Autodesk Fusion 360 part; units mm, degrees
(part 3 of 5)
  spline S30 degree 5 poles (2.192, 23.3898) (2.1931, 23.4016) (2.195, 23.4251) (2.1969, 23.4604) (2.1976, 23.5076) (2.1961, 23.5666) (2.1928, 23.6257) (2.1885, 23.6849) (2.1835, 23.7441) (2.1781, 23.8033) (2.1724, 23.8626) (2.166, 23.9218) (2.159, 23.9811) (2.151, 24.0404) (2.1423, 24.0996) (2.1327, 24.1589) (2.1224, 24.2182) (2.1116, 24.2775) (2.1003, 24.3368) (2.0885, 24.396) (2.0763, 24.4553) (2.0635, 24.5145) (2.0503, 24.5737) (2.0365, 24.6329) (2.0221, 24.6921) (2.0073, 24.7513) (1.992, 24.8104) (1.9762, 24.8696) (1.96, 24.9287) (1.9433, 24.9877) (1.9262, 25.0468) (1.9087, 25.1058) (1.8908, 25.1648) (1.8724, 25.2237) (1.8536, 25.2826) (1.8344, 25.3415) (1.8148, 25.4004) (1.7947, 25.4592) (1.7743, 25.518) (1.7535, 25.5767) (1.7323, 25.6354) (1.7108, 25.694) (1.6888, 25.7526) (1.6665, 25.8112) (1.6438, 25.8697) (1.6207, 25.9282) (1.5972, 25.9866) (1.5734, 26.045) (1.5493, 26.1034) (1.5248, 26.1616) (1.4999, 26.2199) (1.4747, 26.2781) (1.4491, 26.3362) (1.4232, 26.3943) (1.3969, 26.4523) (1.3704, 26.5102) (1.3434, 26.5682) (1.3162, 26.626) (1.2886, 26.6838) (1.2606, 26.7415) (1.2324, 26.7992) (1.2038, 26.8568) (1.1749, 26.9144) (1.1457, 26.9719) (1.1161, 27.0293) (1.0863, 27.0866) (1.0561, 27.1439) (1.0256, 27.2012) (0.9948, 27.2583) (0.9637, 27.3154) (0.9323, 27.3725) (0.9069, 27.418) (0.8877, 27.4522) (0.8749, 27.4749) (0.8685, 27.4863) knots 0 0 0 0 0 0 0.01428571 0.02857143 0.04285714 0.05714286 0.07142857 0.08571429 0.1 0.11428571 0.12857143 0.14285714 0.15714286 0.17142857 0.18571429 0.2 0.21428571 0.22857143 0.24285714 0.25714286 0.27142857 0.28571429 0.3 0.31428571 0.32857143 0.34285714 0.35714286 0.37142857 0.38571429 0.4 0.41428571 0.42857143 0.44285714 0.45714286 0.47142857 0.48571429 0.5 0.51428571 0.52857143 0.54285714 0.55714286 0.57142857 0.58571429 0.6 0.61428571 0.62857143 0.64285714 0.65714286 0.67142857 0.68571429 0.7 0.71428571 0.72857143 0.74285714 0.75714286 0.77142857 0.78571429 0.8 0.81428571 0.82857143 0.84285714 0.85714286 0.87142857 0.88571429 0.9 0.91428571 0.92857143 0.94285714 0.95714286 0.97142857 0.98571429 1 1 1 1 1 1
  arc A62 (0.8685, 27.4863) -> (-0.8685, 27.4863) centre (0, 0) ccw
  spline S31 degree 5 poles (-0.8685, 27.4863) (-0.8749, 27.4749) (-0.8877, 27.4522) (-0.9069, 27.418) (-0.9323, 27.3725) (-0.9637, 27.3154) (-0.9948, 27.2583) (-1.0256, 27.2012) (-1.0561, 27.1439) (-1.0863, 27.0866) (-1.1161, 27.0293) (-1.1457, 26.9719) (-1.1749, 26.9144) (-1.2038, 26.8568) (-1.2324, 26.7992) (-1.2606, 26.7415) (-1.2886, 26.6838) (-1.3162, 26.626) (-1.3434, 26.5682) (-1.3704, 26.5102) (-1.3969, 26.4523) (-1.4232, 26.3943) (-1.4491, 26.3362) (-1.4747, 26.2781) (-1.4999, 26.2199) (-1.5248, 26.1616) (-1.5493, 26.1034) (-1.5734, 26.045) (-1.5972, 25.9866) (-1.6207, 25.9282) (-1.6438, 25.8697) (-1.6665, 25.8112) (-1.6888, 25.7526) (-1.7108, 25.694) (-1.7323, 25.6354) (-1.7535, 25.5767) (-1.7743, 25.518) (-1.7947, 25.4592) (-1.8148, 25.4004) (-1.8344, 25.3415) (-1.8536, 25.2826) (-1.8724, 25.2237) (-1.8908, 25.1648) (-1.9087, 25.1058) (-1.9262, 25.0468) (-1.9433, 24.9877) (-1.96, 24.9287) (-1.9762, 24.8696) (-1.992, 24.8104) (-2.0073, 24.7513) (-2.0221, 24.6921) (-2.0365, 24.6329) (-2.0503, 24.5737) (-2.0635, 24.5145) (-2.0763, 24.4553) (-2.0885, 24.396) (-2.1003, 24.3368) (-2.1116, 24.2775) (-2.1224, 24.2182) (-2.1327, 24.1589) (-2.1423, 24.0996) (-2.151, 24.0404) (-2.159, 23.9811) (-2.166, 23.9218) (-2.1724, 23.8626) (-2.1781, 23.8033) (-2.1835, 23.7441) (-2.1885, 23.6849) (-2.1928, 23.6257) (-2.1961, 23.5666) (-2.1976, 23.5076) (-2.1969, 23.4604) (-2.195, 23.4251) (-2.1931, 23.4016) (-2.192, 23.3898) knots -1 -1 -1 -1 -1 -1 -0.98571429 -0.97142857 -0.95714286 -0.94285714 -0.92857143 -0.91428571 -0.9 -0.88571429 -0.87142857 -0.85714286 -0.84285714 -0.82857143 -0.81428571 -0.8 -0.78571429 -0.77142857 -0.75714286 -0.74285714 -0.72857143 -0.71428571 -0.7 -0.68571429 -0.67142857 -0.65714286 -0.64285714 -0.62857143 -0.61428571 -0.6 -0.58571429 -0.57142857 -0.55714286 -0.54285714 -0.52857143 -0.51428571 -0.5 -0.48571429 -0.47142857 -0.45714286 -0.44285714 -0.42857143 -0.41428571 -0.4 -0.38571429 -0.37142857 -0.35714286 -0.34285714 -0.32857143 -0.31428571 -0.3 -0.28571429 -0.27142857 -0.25714286 -0.24285714 -0.22857143 -0.21428571 -0.2 -0.18571429 -0.17142857 -0.15714286 -0.14285714 -0.12857143 -0.11428571 -0.1 -0.08571429 -0.07142857 -0.05714286 -0.04285714 -0.02857143 -0.01428571 0 0 0 0 0 0
  line L31 (-2.192, 23.3898) -> (-2.1396, 22.8267)
  arc A63 (-2.9987, 21.7434) -> (-2.1396, 22.8267) centre (-3.1353, 22.734) ccw
  arc A64 (-2.9987, 21.7434) -> (-3.8672, 21.6058) centre (0, 0) ccw
  arc A65 (-5.019, 22.3707) -> (-3.8672, 21.6058) centre (-4.0434, 22.5902) ccw
  line L32 (-5.019, 22.3707) -> (-5.1431, 22.9224)
  spline S32 degree 5 poles (-5.1431, 22.9224) (-5.1457, 22.9339) (-5.1512, 22.9569) (-5.1603, 22.9911) (-5.1742, 23.0361) (-5.1939, 23.0918) (-5.2153, 23.147) (-5.2377, 23.2019) (-5.2607, 23.2567) (-5.2841, 23.3114) (-5.3079, 23.3659) (-5.3322, 23.4203) (-5.3573, 23.4745) (-5.3831, 23.5284) (-5.4098, 23.5821) (-5.4372, 23.6355) (-5.4653, 23.6888) (-5.4939, 23.7418) (-5.523, 23.7947) (-5.5525, 23.8474) (-5.5824, 23.9) (-5.6129, 23.9523) (-5.6438, 24.0046) (-5.6752, 24.0566) (-5.7071, 24.1085) (-5.7395, 24.1602) (-5.7724, 24.2117) (-5.8056, 24.263) (-5.8393, 24.3142) (-5.8734, 24.3653) (-5.9079, 24.4161) (-5.9428, 24.4668) (-5.9781, 24.5174) (-6.0138, 24.5678) (-6.0499, 24.618) (-6.0864, 24.6681) (-6.1232, 24.718) (-6.1604, 24.7677) (-6.198, 24.8173) (-6.2359, 24.8667) (-6.2742, 24.916) (-6.3129, 24.9651) (-6.3519, 25.0141) (-6.3912, 25.0629) (-6.4309, 25.1115) (-6.4709, 25.16) (-6.5112, 25.2083) (-6.5519, 25.2565) (-6.5929, 25.3045) (-6.6343, 25.3524) (-6.6759, 25.4001) (-6.7179, 25.4476) (-6.7601, 25.495) (-6.8027, 25.5422) (-6.8456, 25.5893) (-6.8888, 25.6362) (-6.9323, 25.683) (-6.9761, 25.7296) (-7.0202, 25.776) (-7.0646, 25.8223) (-7.1093, 25.8684) (-7.1543, 25.9144) (-7.1996, 25.9602) (-7.2452, 26.0058) (-7.291, 26.0513) (-7.3371, 26.0966) (-7.3835, 26.1418) (-7.4302, 26.1868) (-7.4772, 26.2316) (-7.5244, 26.2763) (-7.5719, 26.3208) (-7.6101, 26.3563) (-7.6389, 26.3829) (-7.6581, 26.4006) (-7.6678, 26.4094) knots 0 0 0 0 0 0 0.01428571 0.02857143 0.04285714 0.05714286 0.07142857 0.08571429 0.1 0.11428571 0.12857143 0.14285714 0.15714286 0.17142857 0.18571429 0.2 0.21428571 0.22857143 0.24285714 0.25714286 0.27142857 0.28571429 0.3 0.31428571 0.32857143 0.34285714 0.35714286 0.37142857 0.38571429 0.4 0.41428571 0.42857143 0.44285714 0.45714286 0.47142857 0.48571429 0.5 0.51428571 0.52857143 0.54285714 0.55714286 0.57142857 0.58571429 0.6 0.61428571 0.62857143 0.64285714 0.65714286 0.67142857 0.68571429 0.7 0.71428571 0.72857143 0.74285714 0.75714286 0.77142857 0.78571429 0.8 0.81428571 0.82857143 0.84285714 0.85714286 0.87142857 0.88571429 0.9 0.91428571 0.92857143 0.94285714 0.95714286 0.97142857 0.98571429 1 1 1 1 1 1
  arc A66 (-7.6678, 26.4094) -> (-9.3197, 25.8726) centre (0, 0) ccw
  spline S33 degree 5 poles (-9.3197, 25.8726) (-9.3223, 25.8598) (-9.3275, 25.8342) (-9.3352, 25.7958) (-9.3452, 25.7447) (-9.3575, 25.6807) (-9.3694, 25.6168) (-9.381, 25.5529) (-9.3924, 25.4891) (-9.4033, 25.4253) (-9.414, 25.3615) (-9.4244, 25.2977) (-9.4344, 25.234) (-9.4441, 25.1704) (-9.4535, 25.1067) (-9.4625, 25.0432) (-9.4712, 24.9796) (-9.4796, 24.9161) (-9.4877, 24.8527) (-9.4954, 24.7893) (-9.5028, 24.7259) (-9.5098, 24.6626) (-9.5165, 24.5994) (-9.5229, 24.5362) (-9.5289, 24.4731) (-9.5345, 24.41) (-9.5398, 24.347) (-9.5448, 24.2841) (-9.5494, 24.2212) (-9.5536, 24.1584) (-9.5575, 24.0956) (-9.561, 24.033) (-9.5642, 23.9704) (-9.5669, 23.9078) (-9.5693, 23.8454) (-9.5713, 23.783) (-9.573, 23.7207) (-9.5742, 23.6585) (-9.5751, 23.5964) (-9.5756, 23.5344) (-9.5756, 23.4724) (-9.5753, 23.4106) (-9.5746, 23.3488) (-9.5734, 23.2872) (-9.5718, 23.2257) (-9.5698, 23.1642) (-9.5674, 23.1029) (-9.5646, 23.0417) (-9.5613, 22.9806) (-9.5576, 22.9196) (-9.5535, 22.8587) (-9.5488, 22.798) (-9.5436, 22.7374) (-9.5379, 22.677) (-9.5318, 22.6167) (-9.5251, 22.5566) (-9.518, 22.4966) (-9.5104, 22.4367) (-9.5024, 22.377) (-9.4938, 22.3175) (-9.4846, 22.2581) (-9.4746, 22.199) (-9.4638, 22.1402) (-9.4523, 22.0817) (-9.44, 22.0233) (-9.4272, 21.9652) (-9.414, 21.9072) (-9.4004, 21.8494) (-9.3863, 21.7918) (-9.3711, 21.7346) (-9.3543, 21.6779) (-9.339, 21.6333) (-9.3263, 21.6003) (-9.3173, 21.5785) (-9.3126, 21.5677) knots -1 -1 -1 -1 -1 -1 -0.98571429 -0.97142857 -0.95714286 -0.94285714 -0.92857143 -0.91428571 -0.9 -0.88571429 -0.87142857 -0.85714286 -0.84285714 -0.82857143 -0.81428571 -0.8 -0.78571429 -0.77142857 -0.75714286 -0.74285714 -0.72857143 -0.71428571 -0.7 -0.68571429 -0.67142857 -0.65714286 -0.64285714 -0.62857143 -0.61428571 -0.6 -0.58571429 -0.57142857 -0.55714286 -0.54285714 -0.52857143 -0.51428571 -0.5 -0.48571429 -0.47142857 -0.45714286 -0.44285714 -0.42857143 -0.41428571 -0.4 -0.38571429 -0.37142857 -0.35714286 -0.34285714 -0.32857143 -0.31428571 -0.3 -0.28571429 -0.27142857 -0.25714286 -0.24285714 -0.22857143 -0.21428571 -0.2 -0.18571429 -0.17142857 -0.15714286 -0.14285714 -0.12857143 -0.11428571 -0.1 -0.08571429 -0.07142857 -0.05714286 -0.04285714 -0.02857143 -0.01428571 0 0 0 0 0 0
  line L33 (-9.3126, 21.5677) -> (-9.0887, 21.0483)
  arc A67 (-9.571, 19.7526) -> (-9.0887, 21.0483) centre (-10.007, 20.6525) ccw
  arc A68 (-9.571, 19.7526) -> (-10.3545, 19.3534) centre (0, 0) ccw
  arc A69 (-11.6862, 19.7248) -> (-10.3545, 19.3534) centre (-10.8262, 20.2351) ccw
  line L34 (-11.6862, 19.7248) -> (-11.9748, 20.2112)
  spline S34 degree 5 poles (-11.9748, 20.2112) (-11.9808, 20.2214) (-11.9931, 20.2415) (-12.0124, 20.2712) (-12.0395, 20.3098) (-12.0754, 20.3566) (-12.1128, 20.4025) (-12.1511, 20.4478) (-12.1899, 20.4928) (-12.2291, 20.5376) (-12.2686, 20.5821) (-12.3085, 20.6263) (-12.3491, 20.6701) (-12.3903, 20.7134) (-12.4323, 20.7562) (-12.4749, 20.7985) (-12.518, 20.8405) (-12.5616, 20.8821) (-12.6056, 20.9234) (-12.65, 20.9644) (-12.6947, 21.0051) (-12.7398, 21.0456) (-12.7854, 21.0857) (-12.8313, 21.1255) (-12.8777, 21.1649) (-12.9245, 21.2041) (-12.9717, 21.2429) (-13.0192, 21.2815) (-13.0671, 21.3198) (-13.1152, 21.3577) (-13.1638, 21.3955) (-13.2126, 21.4329) (-13.2618, 21.4701) (-13.3113, 21.507) (-13.3612, 21.5436) (-13.4113, 21.5799) (-13.4618, 21.616) (-13.5126, 21.6518) (-13.5636, 21.6874) (-13.615, 21.7227) (-13.6666, 21.7577) (-13.7185, 21.7925) (-13.7708, 21.827) (-13.8233, 21.8612) (-13.876, 21.8952) (-13.9291, 21.929) (-13.9824, 21.9625) (-14.0359, 21.9957) (-14.0898, 22.0287) (-14.1439, 22.0615) (-14.1982, 22.0939) (-14.2528, 22.1262) (-14.3077, 22.1582) (-14.3628, 22.1899) (-14.4181, 22.2215) (-14.4737, 22.2527) (-14.5295, 22.2837) (-14.5856, 22.3145) (-14.6419, 22.345) (-14.6984, 22.3753) (-14.7552, 22.4054) (-14.8121, 22.4352) (-14.8694, 22.4648) (-14.9268, 22.4941) (-14.9844, 22.5232) (-15.0423, 22.5521) (-15.1004, 22.5807) (-15.1587, 22.6091) (-15.2172, 22.6372) (-15.276, 22.6651) (-15.3349, 22.6928) (-15.3822, 22.7147) (-15.4178, 22.7311) (-15.4415, 22.7419) (-15.4534, 22.7473) knots 0 0 0 0 0 0 0.01428571 0.02857143 0.04285714 0.05714286 0.07142857 0.08571429 0.1 0.11428571 0.12857143 0.14285714 0.15714286 0.17142857 0.18571429 0.2 0.21428571 0.22857143 0.24285714 0.25714286 0.27142857 0.28571429 0.3 0.31428571 0.32857143 0.34285714 0.35714286 0.37142857 0.38571429 0.4 0.41428571 0.42857143 0.44285714 0.45714286 0.47142857 0.48571429 0.5 0.51428571 0.52857143 0.54285714 0.55714286 0.57142857 0.58571429 0.6 0.61428571 0.62857143 0.64285714 0.65714286 0.67142857 0.68571429 0.7 0.71428571 0.72857143 0.74285714 0.75714286 0.77142857 0.78571429 0.8 0.81428571 0.82857143 0.84285714 0.85714286 0.87142857 0.88571429 0.9 0.91428571 0.92857143 0.94285714 0.95714286 0.97142857 0.98571429 1 1 1 1 1 1
  arc A70 (-15.4534, 22.7473) -> (-16.8586, 21.7264) centre (0, 0) ccw
  spline S35 degree 5 poles (-16.8586, 21.7264) (-16.8572, 21.7134) (-16.8542, 21.6875) (-16.8496, 21.6486) (-16.8434, 21.5968) (-16.8353, 21.5322) (-16.8269, 21.4677) (-16.8182, 21.4034) (-16.8092, 21.3392) (-16.7999, 21.2751) (-16.7904, 21.2111) (-16.7805, 21.1473) (-16.7704, 21.0836) (-16.7599, 21.02) (-16.7492, 20.9566) (-16.7382, 20.8934) (-16.7268, 20.8302) (-16.7152, 20.7673) (-16.7032, 20.7044) (-16.691, 20.6418) (-16.6784, 20.5792) (-16.6656, 20.5169) (-16.6524, 20.4547) (-16.6389, 20.3926) (-16.6251, 20.3307) (-16.611, 20.269) (-16.5966, 20.2074) (-16.5818, 20.146) (-16.5668, 20.0848) (-16.5514, 20.0238) (-16.5357, 19.9629) (-16.5197, 19.9022) (-16.5033, 19.8417) (-16.4866, 19.7814) (-16.4696, 19.7212) (-16.4522, 19.6613) (-16.4345, 19.6015) (-16.4165, 19.542) (-16.3981, 19.4826) (-16.3794, 19.4235) (-16.3604, 19.3646) (-16.3409, 19.3059) (-16.3211, 19.2474) (-16.301, 19.1891) (-16.2805, 19.1311) (-16.2596, 19.0732) (-16.2383, 19.0157) (-16.2167, 18.9583) (-16.1948, 18.9012) (-16.1724, 18.8444) (-16.1496, 18.7878) (-16.1264, 18.7315) (-16.1028, 18.6754) (-16.0787, 18.6197) (-16.0542, 18.5643) (-16.0293, 18.5092) (-16.004, 18.4543) (-15.9783, 18.3997) (-15.9522, 18.3454) (-15.9256, 18.2914) (-15.8985, 18.2378) (-15.8708, 18.1847) (-15.8424, 18.1321) (-15.8132, 18.08) (-15.7835, 18.0283) (-15.7534, 17.977) (-15.7229, 17.9259) (-15.6921, 17.8751) (-15.6609, 17.8247) (-15.6288, 17.775) (-15.5953, 17.7263) (-15.567, 17.6886) (-15.5447, 17.6611) (-15.5294, 17.6432) (-15.5216, 17.6343) knots -1 -1 -1 -1 -1 -1 -0.98571429 -0.97142857 -0.95714286 -0.94285714 -0.92857143 -0.91428571 -0.9 -0.88571429 -0.87142857 -0.85714286 -0.84285714 -0.82857143 -0.81428571 -0.8 -0.78571429 -0.77142857 -0.75714286 -0.74285714 -0.72857143 -0.71428571 -0.7 -0.68571429 -0.67142857 -0.65714286 -0.64285714 -0.62857143 -0.61428571 -0.6 -0.58571429 -0.57142857 -0.55714286 -0.54285714 -0.52857143 -0.51428571 -0.5 -0.48571429 -0.47142857 -0.45714286 -0.44285714 -0.42857143 -0.41428571 -0.4 -0.38571429 -0.37142857 -0.35714286 -0.34285714 -0.32857143 -0.31428571 -0.3 -0.28571429 -0.27142857 -0.25714286 -0.24285714 -0.22857143 -0.21428571 -0.2 -0.18571429 -0.17142857 -0.15714286 -0.14285714 -0.12857143 -0.11428571 -0.1 -0.08571429 -0.07142857 -0.05714286 -0.04285714 -0.02857143 -0.01428571 0 0 0 0 0 0
  line L35 (-15.5216, 17.6343) -> (-15.1482, 17.2096)
  arc A71 (-15.2064, 15.8282) -> (-15.1482, 17.2096) centre (-15.8992, 16.5493) ccw
  arc A72 (-15.2064, 15.8282) -> (-15.8282, 15.2064) centre (0, 0) ccw
  arc A73 (-17.2096, 15.1482) -> (-15.8282, 15.2064) centre (-16.5493, 15.8992) ccw
  line L36 (-17.2096, 15.1482) -> (-17.6343, 15.5216)
  spline S36 degree 5 poles (-17.6343, 15.5216) (-17.6432, 15.5294) (-17.6611, 15.5447) (-17.6886, 15.567) (-17.7263, 15.5953) (-17.775, 15.6288) (-17.8247, 15.6609) (-17.8751, 15.6921) (-17.9259, 15.7229) (-17.977, 15.7534) (-18.0283, 15.7835) (-18.08, 15.8132) (-18.1321, 15.8424) (-18.1847, 15.8708) (-18.2378, 15.8985) (-18.2914, 15.9256) (-18.3454, 15.9522) (-18.3997, 15.9783) (-18.4543, 16.004) (-18.5092, 16.0293) (-18.5643, 16.0542) (-18.6197, 16.0787) (-18.6754, 16.1028) (-18.7315, 16.1264) (-18.7878, 16.1496) (-18.8444, 16.1724) (-18.9012, 16.1948) (-18.9583, 16.2167) (-19.0157, 16.2383) (-19.0732, 16.2596) (-19.1311, 16.2805) (-19.1891, 16.301) (-19.2474, 16.3211) (-19.3059, 16.3409) (-19.3646, 16.3604) (-19.4235, 16.3794) (-19.4826, 16.3981) (-19.542, 16.4165) (-19.6015, 16.4345) (-19.6613, 16.4522) (-19.7212, 16.4696) (-19.7814, 16.4866) (-19.8417, 16.5033) (-19.9022, 16.5197) (-19.9629, 16.5357) (-20.0238, 16.5514) (-20.0848, 16.5668) (-20.146, 16.5818) (-20.2074, 16.5966) (-20.269, 16.611) (-20.3307, 16.6251) (-20.3926, 16.6389) (-20.4547, 16.6524) (-20.5169, 16.6656) (-20.5792, 16.6784) (-20.6418, 16.691) (-20.7044, 16.7032) (-20.7673, 16.7152) (-20.8302, 16.7268) (-20.8934, 16.7382) (-20.9566, 16.7492) (-21.02, 16.7599) (-21.0836, 16.7704) (-21.1473, 16.7805) (-21.2111, 16.7904) (-21.2751, 16.7999) (-21.3392, 16.8092) (-21.4034, 16.8182) (-21.4677, 16.8269) (-21.5322, 16.8353) (-21.5968, 16.8434) (-21.6486, 16.8496) (-21.6875, 16.8542) (-21.7134, 16.8572) (-21.7264, 16.8586) knots 0 0 0 0 0 0 0.01428571 0.02857143 0.04285714 0.05714286 0.07142857 0.08571429 0.1 0.11428571 0.12857143 0.14285714 0.15714286 0.17142857 0.18571429 0.2 0.21428571 0.22857143 0.24285714 0.25714286 0.27142857 0.28571429 0.3 0.31428571 0.32857143 0.34285714 0.35714286 0.37142857 0.38571429 0.4 0.41428571 0.42857143 0.44285714 0.45714286 0.47142857 0.48571429 0.5 0.51428571 0.52857143 0.54285714 0.55714286 0.57142857 0.58571429 0.6 0.61428571 0.62857143 0.64285714 0.65714286 0.67142857 0.68571429 0.7 0.71428571 0.72857143 0.74285714 0.75714286 0.77142857 0.78571429 0.8 0.81428571 0.82857143 0.84285714 0.85714286 0.87142857 0.88571429 0.9 0.91428571 0.92857143 0.94285714 0.95714286 0.97142857 0.98571429 1 1 1 1 1 1
  arc A74 (-21.7264, 16.8586) -> (-22.7473, 15.4534) centre (0, 0) ccw
  spline S37 degree 5 poles (-22.7473, 15.4534) (-22.7419, 15.4415) (-22.7311, 15.4178) (-22.7147, 15.3822) (-22.6928, 15.3349) (-22.6651, 15.276) (-22.6372, 15.2172) (-22.6091, 15.1587) (-22.5807, 15.1004) (-22.5521, 15.0423) (-22.5232, 14.9844) (-22.4941, 14.9268) (-22.4648, 14.8694) (-22.4352, 14.8121) (-22.4054, 14.7552) (-22.3753, 14.6984) (-22.345, 14.6419) (-22.3145, 14.5856) (-22.2837, 14.5295) (-22.2527, 14.4737) (-22.2215, 14.4181) (-22.1899, 14.3628) (-22.1582, 14.3077) (-22.1262, 14.2528) (-22.0939, 14.1982) (-22.0615, 14.1439) (-22.0287, 14.0898) (-21.9957, 14.0359) (-21.9625, 13.9824) (-21.929, 13.9291) (-21.8952, 13.876) (-21.8612, 13.8233) (-21.827, 13.7708) (-21.7925, 13.7185) (-21.7577, 13.6666) (-21.7227, 13.615) (-21.6874, 13.5636) (-21.6518, 13.5126) (-21.616, 13.4618) (-21.5799, 13.4113) (-21.5436, 13.3612) (-21.507, 13.3113) (-21.4701, 13.2618) (-21.4329, 13.2126) (-21.3955, 13.1638) (-21.3577, 13.1152) (-21.3198, 13.0671) (-21.2815, 13.0192) (-21.2429, 12.9717) (-21.2041, 12.9245) (-21.1649, 12.8777) (-21.1255, 12.8313) (-21.0857, 12.7854) (-21.0456, 12.7398) (-21.0051, 12.6947) (-20.9644, 12.65) (-20.9234, 12.6056) (-20.8821, 12.5616) (-20.8405, 12.518) (-20.7985, 12.4749) (-20.7562, 12.4323) (-20.7134, 12.3903) (-20.6701, 12.3491) (-20.6263, 12.3085) (-20.5821, 12.2686) (-20.5376, 12.2291) (-20.4928, 12.1899) (-20.4478, 12.1511) (-20.4025, 12.1128) (-20.3566, 12.0754) (-20.3098, 12.0395) (-20.2712, 12.0124) (-20.2415, 11.9931) (-20.2214, 11.9808) (-20.2112, 11.9748) knots -1 -1 -1 -1 -1 -1 -0.98571429 -0.97142857 -0.95714286 -0.94285714 -0.92857143 -0.91428571 -0.9 -0.88571429 -0.87142857 -0.85714286 -0.84285714 -0.82857143 -0.81428571 -0.8 -0.78571429 -0.77142857 -0.75714286 -0.74285714 -0.72857143 -0.71428571 -0.7 -0.68571429 -0.67142857 -0.65714286 -0.64285714 -0.62857143 -0.61428571 -0.6 -0.58571429 -0.57142857 -0.55714286 -0.54285714 -0.52857143 -0.51428571 -0.5 -0.48571429 -0.47142857 -0.45714286 -0.44285714 -0.42857143 -0.41428571 -0.4 -0.38571429 -0.37142857 -0.35714286 -0.34285714 -0.32857143 -0.31428571 -0.3 -0.28571429 -0.27142857 -0.25714286 -0.24285714 -0.22857143 -0.21428571 -0.2 -0.18571429 -0.17142857 -0.15714286 -0.14285714 -0.12857143 -0.11428571 -0.1 -0.08571429 -0.07142857 -0.05714286 -0.04285714 -0.02857143 -0.01428571 0 0 0 0 0 0
  line L37 (-20.2112, 11.9748) -> (-19.7248, 11.6862)
  arc A75 (-19.3534, 10.3545) -> (-19.7248, 11.6862) centre (-20.2351, 10.8262) ccw
  arc A76 (-19.3534, 10.3545) -> (-19.7526, 9.571) centre (0, 0) ccw
  arc A77 (-21.0483, 9.0887) -> (-19.7526, 9.571) centre (-20.6525, 10.007) ccw
  line L38 (-21.0483, 9.0887) -> (-21.5677, 9.3126)
  spline S38 degree 5 poles (-21.5677, 9.3126) (-21.5785, 9.3173) (-21.6003, 9.3263) (-21.6333, 9.339) (-21.6779, 9.3543) (-21.7346, 9.3711) (-21.7918, 9.3863) (-21.8494, 9.4004) (-21.9072, 9.414) (-21.9652, 9.4272) (-22.0233, 9.44) (-22.0817, 9.4523) (-22.1402, 9.4638) (-22.199, 9.4746) (-22.2581, 9.4846) (-22.3175, 9.4938) (-22.377, 9.5024) (-22.4367, 9.5104) (-22.4966, 9.518) (-22.5566, 9.5251) (-22.6167, 9.5318) (-22.677, 9.5379) (-22.7374, 9.5436) (-22.798, 9.5488) (-22.8587, 9.5535) (-22.9196, 9.5576) (-22.9806, 9.5613) (-23.0417, 9.5646) (-23.1029, 9.5674) (-23.1642, 9.5698) (-23.2257, 9.5718) (-23.2872, 9.5734) (-23.3488, 9.5746) (-23.4106, 9.5753) (-23.4724, 9.5756) (-23.5344, 9.5756) (-23.5964, 9.5751) (-23.6585, 9.5742) (-23.7207, 9.573) (-23.783, 9.5713) (-23.8454, 9.5693) (-23.9078, 9.5669) (-23.9704, 9.5642) (-24.033, 9.561) (-24.0956, 9.5575) (-24.1584, 9.5536) (-24.2212, 9.5494) (-24.2841, 9.5448) (-24.347, 9.5398) (-24.41, 9.5345) (-24.4731, 9.5289) (-24.5362, 9.5229) (-24.5994, 9.5165) (-24.6626, 9.5098) (-24.7259, 9.5028) (-24.7893, 9.4954) (-24.8527, 9.4877) (-24.9161, 9.4796) (-24.9796, 9.4712) (-25.0432, 9.4625) (-25.1067, 9.4535) (-25.1704, 9.4441) (-25.234, 9.4344) (-25.2977, 9.4244) (-25.3615, 9.414) (-25.4253, 9.4033) (-25.4891, 9.3924) (-25.5529, 9.381) (-25.6168, 9.3694) (-25.6807, 9.3575) (-25.7447, 9.3452) (-25.7958, 9.3352) (-25.8342, 9.3275) (-25.8598, 9.3223) (-25.8726, 9.3197) knots 0 0 0 0 0 0 0.01428571 0.02857143 0.04285714 0.05714286 0.07142857 0.08571429 0.1 0.11428571 0.12857143 0.14285714 0.15714286 0.17142857 0.18571429 0.2 0.21428571 0.22857143 0.24285714 0.25714286 0.27142857 0.28571429 0.3 0.31428571 0.32857143 0.34285714 0.35714286 0.37142857 0.38571429 0.4 0.41428571 0.42857143 0.44285714 0.45714286 0.47142857 0.48571429 0.5 0.51428571 0.52857143 0.54285714 0.55714286 0.57142857 0.58571429 0.6 0.61428571 0.62857143 0.64285714 0.65714286 0.67142857 0.68571429 0.7 0.71428571 0.72857143 0.74285714 0.75714286 0.77142857 0.78571429 0.8 0.81428571 0.82857143 0.84285714 0.85714286 0.87142857 0.88571429 0.9 0.91428571 0.92857143 0.94285714 0.95714286 0.97142857 0.98571429 1 1 1 1 1 1
  arc A78 (-25.8726, 9.3197) -> (-26.4094, 7.6678) centre (0, 0) ccw
  spline S39 degree 5 poles (-26.4094, 7.6678) (-26.4006, 7.6581) (-26.3829, 7.6389) (-26.3563, 7.6101) (-26.3208, 7.5719) (-26.2763, 7.5244) (-26.2316, 7.4772) (-26.1868, 7.4302) (-26.1418, 7.3835) (-26.0966, 7.3371) (-26.0513, 7.291) (-26.0058, 7.2452) (-25.9602, 7.1996) (-25.9144, 7.1543) (-25.8684, 7.1093) (-25.8223, 7.0646) (-25.776, 7.0202) (-25.7296, 6.9761) (-25.683, 6.9323) (-25.6362, 6.8888) (-25.5893, 6.8456) (-25.5422, 6.8027) (-25.495, 6.7601) (-25.4476, 6.7179) (-25.4001, 6.6759) (-25.3524, 6.6343) (-25.3045, 6.5929) (-25.2565, 6.5519) (-25.2083, 6.5112) (-25.16, 6.4709) (-25.1115, 6.4309) (-25.0629, 6.3912) (-25.0141, 6.3519) (-24.9651, 6.3129) (-24.916, 6.2742) (-24.8667, 6.2359) (-24.8173, 6.198) (-24.7677, 6.1604) (-24.718, 6.1232) (-24.6681, 6.0864) (-24.618, 6.0499) (-24.5678, 6.0138) (-24.5174, 5.9781) (-24.4668, 5.9428) (-24.4161, 5.9079) (-24.3653, 5.8734) (-24.3142, 5.8393) (-24.263, 5.8056) (-24.2117, 5.7724) (-24.1602, 5.7395) (-24.1085, 5.7071) (-24.0566, 5.6752) (-24.0046, 5.6438) (-23.9523, 5.6129) (-23.9, 5.5824) (-23.8474, 5.5525) (-23.7947, 5.523) (-23.7418, 5.4939) (-23.6888, 5.4653) (-23.6355, 5.4372) (-23.5821, 5.4098) (-23.5284, 5.3831) (-23.4745, 5.3573) (-23.4203, 5.3322) (-23.3659, 5.3079) (-23.3114, 5.2841) (-23.2567, 5.2607) (-23.2019, 5.2377) (-23.147, 5.2153) (-23.0918, 5.1939) (-23.0361, 5.1742) (-22.9911, 5.1603) (-22.9569, 5.1512) (-22.9339, 5.1457) (-22.9224, 5.1431) knots -1 -1 -1 -1 -1 -1 -0.98571429 -0.97142857 -0.95714286 -0.94285714 -0.92857143 -0.91428571 -0.9 -0.88571429 -0.87142857 -0.85714286 -0.84285714 -0.82857143 -0.81428571 -0.8 -0.78571429 -0.77142857 -0.75714286 -0.74285714 -0.72857143 -0.71428571 -0.7 -0.68571429 -0.67142857 -0.65714286 -0.64285714 -0.62857143 -0.61428571 -0.6 -0.58571429 -0.57142857 -0.55714286 -0.54285714 -0.52857143 -0.51428571 -0.5 -0.48571429 -0.47142857 -0.45714286 -0.44285714 -0.42857143 -0.41428571 -0.4 -0.38571429 -0.37142857 -0.35714286 -0.34285714 -0.32857143 -0.31428571 -0.3 -0.28571429 -0.27142857 -0.25714286 -0.24285714 -0.22857143 -0.21428571 -0.2 -0.18571429 -0.17142857 -0.15714286 -0.14285714 -0.12857143 -0.11428571 -0.1 -0.08571429 -0.07142857 -0.05714286 -0.04285714 -0.02857143 -0.01428571 0 0 0 0 0 0
  line L39 (-22.9224, 5.1431) -> (-22.3707, 5.019)
  arc A79 (-21.6058, 3.8672) -> (-22.3707, 5.019) centre (-22.5902, 4.0434) ccw
  circle A80 centre (0, 0) radius 7.5
  circle A81 centre (0, 0) radius 16
  circle A82 centre (0, 0) radius 7.5
  dimension "d8" = 32
  constraint concentric A0 A81
  constraint concentric A81 A82
  measures "d8" diameter of A81
extrude "Extrude3" add sketch "Sketch1 (2)" along normal blind 15 contours A81 in component "Spur Gear (20 teeth)"
component "Spur Gear (20 teeth)" placed x (1, 0, 0) y (0, 1, 0) z (0, 0, 1) at (0, 0, 0)
equation "d9 = 40 mm - 25 mm"

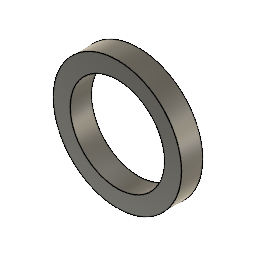
design "entretoise"
Autodesk Fusion 360 part; units mm, degrees
sketch "Sketch1" plane through (0, 0, 0) normal (0, 1, 0) x (1, 0, 0)
  circle A0 centre (0, 0) radius 15
  circle A1 centre (0, 0) radius 11
  dimension "d1" = 30
  dimension "d2" = 22
  constraint coincident A0.centre A1.centre
  measures "d1" diameter of A0
  measures "d2" diameter of A1
extrude "Extrude1" add sketch "Sketch1" along normal blind 5

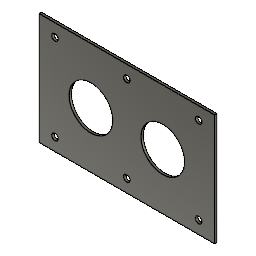
design "cale extérieur"
Autodesk Fusion 360 part; units mm, degrees
sketch "Sketch1" plane through (0, 0, 0) normal (0, 1, 0) x (1, 0, 0)
  line L0 (-88.4437, -50) -> (21.5563, -50)
  line L1 (21.5563, -50) -> (21.5563, 20)
  line L2 (21.5563, 20) -> (-88.4437, 20)
  line L3 (-88.4437, 20) -> (-88.4437, -50)
  line L4 (-88.4437, -15) -> (21.5563, -15) construction
  circle A0 centre (-55.9437, -15) radius 13.6
  circle A1 centre (-10.9437, -15) radius 13.6
  line L5 (-55.9437, -15) -> (-55.9437, -5) construction
  line L6 (-55.9437, -5) -> (-10.9437, -5) construction
  line L7 (-10.9437, -5) -> (-10.9437, -15) construction
  line L8 (-33.4437, -5) -> (-33.4437, -15) construction
  dimension "d1" = 70
  dimension "d2" = 110
  dimension "d3" = 27.2
  dimension "d4" = 45
  constraint horizontal L0
  constraint vertical L1
  constraint horizontal L2
  constraint vertical L3
  constraint midpoint L3 L4.start
  constraint midpoint L1 L4.end
  constraint coincident L4 A0.centre
  constraint coincident L4 A1.centre
  constraint equal A0 A1
  constraint coincident A0.centre L5.start
  constraint perpendicular L4 L5
  constraint perpendicular L5 L6
  constraint perpendicular L6 L7
  constraint coincident A1.centre L7.end
  constraint midpoint L6 L8.start
  constraint perpendicular L6 L8
  constraint midpoint L4 L8.end
  measures "d1" distance of L0.start L2.end
  measures "d2" distance of L0.start L0.end
  measures "d3" diameter of A0
  measures "d4" distance of A0.centre A1.centre L0.start
extrude "Extrude1" add sketch "Sketch1" along normal blind 1.5
sketch "Sketch2" plane through (0, 0, 0) normal (0, -1, 0) x (1, 0, 0)
  circle A0 centre (-10.9437, 15) radius 13.6
  circle A1 centre (-55.9437, 15) radius 13.6
  line L0 (-88.4437, 50) -> (-88.4437, -20)
  line L1 (-88.4437, -20) -> (21.5563, -20)
  line L2 (21.5563, -20) -> (21.5563, 50)
  line L3 (21.5563, 50) -> (-88.4437, 50)
  line L4 (-88.4437, 42) -> (21.5563, 42) construction
  circle A2 centre (-33.4437, 42) radius 2
  circle A3 centre (-78.4437, 42) radius 2
  circle A4 centre (11.5563, 42) radius 2
  line L5 (-88.4437, 15) -> (21.5563, 15) construction
  circle A5 centre (-78.4437, -12) radius 2
  circle A6 centre (-33.4437, -12) radius 2
  circle A7 centre (11.5563, -12) radius 2
  dimension "d7" = 4
  dimension "d8" = 8
  dimension "d9" = 10
  dimension "d10" = 10
  constraint coincident L0 L4.start
  constraint coincident L2 L4.end
  constraint perpendicular L2 L4
  constraint midpoint L4 A2.centre
  constraint coincident L4 A3.centre
  constraint coincident L4 A4.centre
  constraint equal A2 A4
  constraint equal A2 A3
  constraint midpoint L0 L5.start
  constraint midpoint L2 L5.end
  constraint symmetric A2 L5 A6
  constraint symmetric A3 L5 A5
  constraint symmetric A4 L5 A7
  measures "d7" diameter of A3
  measures "d8" distance of L3 L4
  measures "d9" distance of L0 A3.centre
  measures "d10" distance of L2 A4.centre
extrude "Extrude2" cut sketch "Sketch2" against normal through all contours A2 | A3 | A4 | A5 | A6 | A7
equation "d10 = d9"

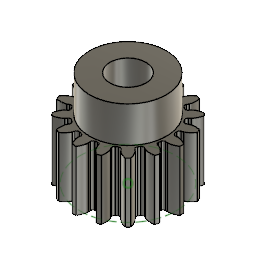
design "Engrenage 16D M2.5"
description: Spur Gear; Module: 2.5; Num Teeth: 16; Pressure Angle: 20.0; Backlash: 0.00 mm
Autodesk Fusion 360 part; units mm, degrees
sketch "Sketch1" plane through (0, 0, 0) normal (0, 0, 1) x (1, 0, 0) in component "Spur Gear (16 teeth)"
  circle A0 centre (0, 0) radius 16.9492
  circle A1 centre (0, 0) radius 7.5
extrude "Extrude1" add sketch "Sketch1" along normal blind 25 in component "Spur Gear (16 teeth)"
sketch "Sketch2" plane through (0, 0, 0) normal (0, 0, 1) x (1, 0, 0) in component "Spur Gear (16 teeth)"
  spline S0 degree 5 poles (18.6738, -2.1207) (18.6847, -2.1219) (18.7065, -2.124) (18.7393, -2.1263) (18.783, -2.1276) (18.8378, -2.1268) (18.8928, -2.1242) (18.9478, -2.1205) (19.0028, -2.1162) (19.0579, -2.1115) (19.113, -2.1064) (19.1681, -2.1008) (19.2232, -2.0944) (19.2784, -2.0871) (19.3336, -2.079) (19.3888, -2.0701) (19.444, -2.0605) (19.4992, -2.0503) (19.5544, -2.0396) (19.6096, -2.0285) (19.6648, -2.0169) (19.72, -2.0048) (19.7752, -1.9921) (19.8303, -1.9789) (19.8855, -1.9652) (19.9406, -1.9509) (19.9957, -1.9362) (20.0508, -1.921) (20.1059, -1.9054) (20.1609, -1.8893) (20.2159, -1.8728) (20.2709, -1.8558) (20.3259, -1.8384) (20.3808, -1.8206) (20.4357, -1.8024) (20.4906, -1.7837) (20.5454, -1.7646) (20.6002, -1.7451) (20.655, -1.7252) (20.7097, -1.7049) (20.7643, -1.6842) (20.819, -1.6631) (20.8736, -1.6416) (20.9281, -1.6198) (20.9826, -1.5975) (21.037, -1.5749) (21.0914, -1.5519) (21.1458, -1.5285) (21.2001, -1.5048) (21.2543, -1.4807) (21.3085, -1.4563) (21.3626, -1.4315) (21.4167, -1.4063) (21.4707, -1.3808) (21.5247, -1.3549) (21.5786, -1.3287) (21.6324, -1.3021) (21.6862, -1.2752) (21.7399, -1.248) (21.7936, -1.2204) (21.8471, -1.1925) (21.9007, -1.1642) (21.9541, -1.1356) (22.0075, -1.1067) (22.0608, -1.0775) (22.114, -1.0479) (22.1672, -1.018) (22.2203, -0.9878) (22.2733, -0.9573) (22.3263, -0.9265) (22.3791, -0.8953) (22.4214, -0.8701) (22.453, -0.8511) (22.4741, -0.8383) (22.4846, -0.8319) knots 0 0 0 0 0 0 0.01428571 0.02857143 0.04285714 0.05714286 0.07142857 0.08571429 0.1 0.11428571 0.12857143 0.14285714 0.15714286 0.17142857 0.18571429 0.2 0.21428571 0.22857143 0.24285714 0.25714286 0.27142857 0.28571429 0.3 0.31428571 0.32857143 0.34285714 0.35714286 0.37142857 0.38571429 0.4 0.41428571 0.42857143 0.44285714 0.45714286 0.47142857 0.48571429 0.5 0.51428571 0.52857143 0.54285714 0.55714286 0.57142857 0.58571429 0.6 0.61428571 0.62857143 0.64285714 0.65714286 0.67142857 0.68571429 0.7 0.71428571 0.72857143 0.74285714 0.75714286 0.77142857 0.78571429 0.8 0.81428571 0.82857143 0.84285714 0.85714286 0.87142857 0.88571429 0.9 0.91428571 0.92857143 0.94285714 0.95714286 0.97142857 0.98571429 1 1 1 1 1 1
  spline S1 degree 5 poles (18.6738, 2.1207) (18.6847, 2.1219) (18.7065, 2.124) (18.7393, 2.1263) (18.783, 2.1276) (18.8378, 2.1268) (18.8928, 2.1242) (18.9478, 2.1205) (19.0028, 2.1162) (19.0579, 2.1115) (19.113, 2.1064) (19.1681, 2.1008) (19.2232, 2.0944) (19.2784, 2.0871) (19.3336, 2.079) (19.3888, 2.0701) (19.444, 2.0605) (19.4992, 2.0503) (19.5544, 2.0396) (19.6096, 2.0285) (19.6648, 2.0169) (19.72, 2.0048) (19.7752, 1.9921) (19.8303, 1.9789) (19.8855, 1.9652) (19.9406, 1.9509) (19.9957, 1.9362) (20.0508, 1.921) (20.1059, 1.9054) (20.1609, 1.8893) (20.2159, 1.8728) (20.2709, 1.8558) (20.3259, 1.8384) (20.3808, 1.8206) (20.4357, 1.8024) (20.4906, 1.7837) (20.5454, 1.7646) (20.6002, 1.7451) (20.655, 1.7252) (20.7097, 1.7049) (20.7643, 1.6842) (20.819, 1.6631) (20.8736, 1.6416) (20.9281, 1.6198) (20.9826, 1.5975) (21.037, 1.5749) (21.0914, 1.5519) (21.1458, 1.5285) (21.2001, 1.5048) (21.2543, 1.4807) (21.3085, 1.4563) (21.3626, 1.4315) (21.4167, 1.4063) (21.4707, 1.3808) (21.5247, 1.3549) (21.5786, 1.3287) (21.6324, 1.3021) (21.6862, 1.2752) (21.7399, 1.248) (21.7936, 1.2204) (21.8471, 1.1925) (21.9007, 1.1642) (21.9541, 1.1356) (22.0075, 1.1067) (22.0608, 1.0775) (22.114, 1.0479) (22.1672, 1.018) (22.2203, 0.9878) (22.2733, 0.9573) (22.3263, 0.9265) (22.3791, 0.8953) (22.4214, 0.8701) (22.453, 0.8511) (22.4741, 0.8383) (22.4846, 0.8319) knots 0 0 0 0 0 0 0.01428571 0.02857143 0.04285714 0.05714286 0.07142857 0.08571429 0.1 0.11428571 0.12857143 0.14285714 0.15714286 0.17142857 0.18571429 0.2 0.21428571 0.22857143 0.24285714 0.25714286 0.27142857 0.28571429 0.3 0.31428571 0.32857143 0.34285714 0.35714286 0.37142857 0.38571429 0.4 0.41428571 0.42857143 0.44285714 0.45714286 0.47142857 0.48571429 0.5 0.51428571 0.52857143 0.54285714 0.55714286 0.57142857 0.58571429 0.6 0.61428571 0.62857143 0.64285714 0.65714286 0.67142857 0.68571429 0.7 0.71428571 0.72857143 0.74285714 0.75714286 0.77142857 0.78571429 0.8 0.81428571 0.82857143 0.84285714 0.85714286 0.87142857 0.88571429 0.9 0.91428571 0.92857143 0.94285714 0.95714286 0.97142857 0.98571429 1 1 1 1 1 1
  arc A0 (22.4846, -0.8319) -> (22.4846, 0.8319) centre (0, 0) ccw
  line L0 (16.831, -1.9125) -> (18.6738, -2.1207)
  line L1 (16.831, 1.9125) -> (18.6738, 2.1207)
  line L2 (16.831, -1.9125) -> (16.831, 1.9125)
  point P0 (18.9402, -2.1209)
  point P1 (19.2093, -2.0959)
  point P2 (19.4801, -2.0538)
  point P3 (19.752, -1.9973)
  point P4 (20.0249, -1.9281)
  point P5 (20.2983, -1.8471)
  point P6 (20.5722, -1.755)
  point P7 (20.8463, -1.6523)
  point P8 (21.1203, -1.5394)
  point P9 (21.3942, -1.4167)
  point P10 (21.6678, -1.2844)
  point P11 (21.9408, -1.1427)
  point P12 (22.2131, -0.9918)
  point P13 (18.9402, 2.1209)
  point P14 (19.2093, 2.0959)
  point P15 (19.4801, 2.0538)
  point P16 (19.752, 1.9973)
  point P17 (20.0249, 1.9281)
  point P18 (20.2983, 1.8471)
  point P19 (20.5722, 1.755)
  point P20 (20.8463, 1.6523)
  point P21 (21.1203, 1.5394)
  point P22 (21.3942, 1.4167)
  point P23 (21.6678, 1.2844)
  point P24 (21.9408, 1.1427)
  point P25 (22.2131, 0.9918)
extrude "Extrude2" add sketch "Sketch2" along normal blind 25 in component "Spur Gear (16 teeth)"
fillet "Fillet1" radius 1 2 edges at (16.8408, -1.9136, 12.5) (16.8408, 1.9136, 12.5) in component "Spur Gear (16 teeth)"
pattern_circular "C-Pattern1" count 16 over 360 about axis through (0, 0, 0) along (0, 0, 1) of "Extrude2", "Fillet1" in component "Spur Gear (16 teeth)"
sketch "Sketch3" plane through (0, 0, 0) normal (0, 0, 1) x (1, 0, 0) in component "Spur Gear (16 teeth)"
  circle A0 centre (0, 0) radius 20 construction